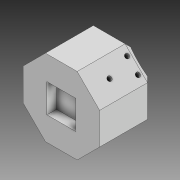
# Autodesk Inventor part: Body
Saved by Autodesk Inventor 2020 (Build 240168000, 168)
## iProperties
Created: 2021-03-26
Part Number: Body
Material: Generic
Document SubType Name: Modeling
Designer: DDeGo
Density: 1 g/cm^3
Appearance: Default
Author: DDeGo
Autodesk Inventor part; units mm, degrees
ref_plane "YZ Plane" through (0, 0, 0) normal (1, 0, 0) x (0, 1, 0)
ref_plane "XZ Plane" through (0, 0, 0) normal (0, 1, 0) x (-1, 0, 0)
ref_plane "XY Plane" through (0, 0, 0) normal (0, 0, 1) x (1, 0, 0)
sketch "Sketch1" plane through (0, 0, 0) normal (0, 0, 1) x (1, 0, 0)
  circle A0 centre (0, 0) radius 16.002 construction
  line L0 (8.2843, 20) -> (20, 8.2843)
  line L1 (20, 8.2843) -> (20, -8.2843)
  line L2 (20, -8.2843) -> (8.2843, -20)
  line L3 (8.2843, -20) -> (-8.2843, -20)
  line L4 (-8.2843, -20) -> (-20, -8.2843)
  line L5 (-20, -8.2843) -> (-20, 8.2843)
  line L6 (-20, 8.2843) -> (-8.2843, 20)
  line L7 (-8.2843, 20) -> (8.2843, 20)
  dimension "d0" = 32.004
  dimension "d2" = 40
  constraints: 16 end point, 3 coincident, 1 centre point, 1 vertical, 17 other
  measures "d0" diameter of A0
  measures "d2" distance between parallel lines of L1 L5
extrude "Extrusion1" add sketch "Sketch1" along normal blind 30
chamfer "Chamfer1" distance 5 angle 45 8 edges at (-14.1421, 14.1421, 0) (-20, 0, 0) (-14.1421, -14.1421, 0) (0, -20, 0) (14.1421, -14.1421, 0) (20, 0, 0) (14.1421, 14.1421, 0) (0, 20, 0)
sketch "Sketch2" plane through (0, 0, 0) normal (0, 0, -1) x (-1, 0, 0)
  circle A0 centre (0, 0) radius 16.002 construction
  circle A1 centre (0, 0) radius 16.302
  dimension "d8" = 32.004
  dimension "d9" = 0.3
  constraints: 2 centre point, 2 coincident
  measures "d8" diameter of A0
  measures "d9" radial gap between concentric circles of A0 A1
extrude "Extrusion2" cut sketch "Sketch2" against normal blind 8
sketch "Sketch4" plane through (0, 0, 30) normal (0, 0, 1) x (1, 0, 0)
  line L0 (-7.5, -7.5) -> (7.5, -7.5)
  line L1 (7.5, -7.5) -> (7.5, 7.5)
  line L2 (7.5, 7.5) -> (-7.5, 7.5)
  line L3 (-7.5, 7.5) -> (-7.5, -7.5)
  line L4 (-7.5, -7.5) -> (7.5, 7.5) construction
  line L5 (7.5, -7.5) -> (-7.5, 7.5) construction
  point P0 (0, 0)
  dimension "d18" = 15
  dimension "d19" = 15
  constraints: 12 end point, 2 midpoint, 2 parallel, 1 horizontal, 1 perpendicular
  measures "d18" distance of L1.end L2.end
  measures "d19" distance of L0.end L1.end
extrude "Extrusion4" cut sketch "Sketch4" against normal blind 5
sketch "Sketch3" plane through (-8.2843, -20, 30) normal (-0.7071, -0.7071, 0) x (-0.7071, 0.7071, 0)
  line L0 (12.2843, 11) -> (4.2843, 11) construction
  line L1 (4.2843, 11) -> (4.2843, 23) construction
  line L2 (4.2843, 23) -> (12.2843, 23) construction
  line L3 (12.2843, 23) -> (12.2843, 11) construction
  line L4 (12.2843, 11) -> (4.2843, 23) construction
  line L5 (4.2843, 11) -> (12.2843, 23) construction
  line L6 (8.2843, 17) -> (8.2843, 30) construction
  circle A0 centre (8.2843, 11) radius 1.15
  circle A1 centre (12.2843, 23) radius 1.15
  circle A2 centre (4.2843, 23) radius 1.15
  dimension "d12" = 13
  dimension "d13" = 12
  dimension "d14" = 8
  dimension "d15" = 2.3
  constraints: 14 end point, 3 centre point, 3 midpoint, 2 coincident, 2 equal radius, 2 parallel, 1 horizontal, 1 perpendicular, 1 vertical
  measures "d12" distance of L6.start L6.end
  measures "d13" distance of L0.end L1.end
  measures "d14" distance of L0.start L0.end
  measures "d15" diameter of A1
extrude "Extrusion3" cut sketch "Sketch3" against normal blind 3
pattern_circular "Circular Pattern1" count 4 over 360 about axis through (0, 0, -10) along (0, 0, 1) of "Extrusion3"
body "Solid1"
